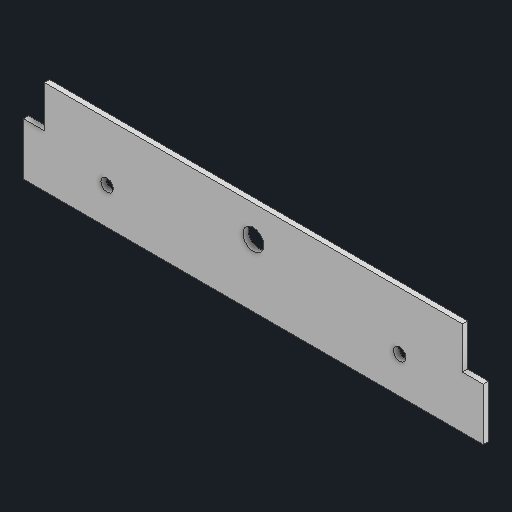
# Autodesk Inventor part: sUPORTE1
Saved by Autodesk Inventor 2026.2 (Build 302298010, 298A)
## iProperties
Created: 2026-02-20
Part Number: sUPORTE1
Material: Generic
Document SubType Name: Modeling
Designer: 062210040
Density: 1 g/cm^3
Appearance: Default
Author: 062210040
Autodesk Inventor part; units mm, degrees
ref_plane "YZ Plane" through (0, 0, 0) normal (1, 0, 0) x (0, 1, 0)
ref_plane "XZ Plane" through (0, 0, 0) normal (0, 1, 0) x (-1, 0, 0)
ref_plane "XY Plane" through (0, 0, 0) normal (0, 0, 1) x (1, 0, 0)
sketch "Sketch1" plane through (0, 0, 0) normal (0, 0, 1) x (1, 0, 0)
  line L0 (0, 0) -> (0, 50)
  line L1 (0, 50) -> (20, 50)
  line L2 (20, 50) -> (20, 90)
  line L3 (20, 90) -> (420, 90)
  line L4 (420, 90) -> (420, 50)
  line L5 (420, 50) -> (440, 50)
  line L6 (440, 50) -> (440, 0)
  line L7 (440, 0) -> (0, 0)
  circle A0 centre (220, 60) radius 10
  circle A1 centre (80, 35) radius 6
  circle A2 centre (360, 35) radius 6
  circle A3 centre (80, 35) radius 50
  circle A4 centre (130, 35) radius 6
  circle A5 centre (310, 35) radius 6
  dimension "d1" = 50
  dimension "d2" = 20
  dimension "d3" = 40
  dimension "d4" = 400
  dimension "d5" = 40
  dimension "d6" = 20
  dimension "d7" = 20
  dimension "d8" = 12
  dimension "d9" = 12
  dimension "d10" = 80
  dimension "d11" = 80
  dimension "d12" = 35
  dimension "d13" = 35
  dimension "d14" = 30
  dimension "d17" = 100
  dimension "d18" = 12
  dimension "d19" = 12
  dimension "d20" = 130
  dimension "d21" = 130
  dimension "d22" = 35
  dimension "d23" = 35
  constraints: 16 end point, 6 centre point, 5 perpendicular, 2 horizontal, 1 coincident, 1 vertical
  measures "d1" distance of L0.start L0.end
  measures "d2" distance of L0.end L1.end
  measures "d3" distance of L1.end L2.end
  measures "d4" distance of L2.end L3.end
  measures "d5" distance of L3.end L4.end
  measures "d6" distance of L4.end L5.end
  measures "d7" diameter of A0
  measures "d8" diameter of A1
  measures "d9" diameter of A2
  measures "d10" distance from line of L6 A2.centre
  measures "d11" distance from line of L0 A1.centre
  measures "d12" distance from line of L7 A1.centre
  measures "d13" distance from line of A2.centre L7
  measures "d14" distance from line of L3 A0.centre
  measures "d17" diameter of A3
  measures "d18" diameter of A4
  measures "d19" diameter of A5
  measures "d20" distance from line of L6 A5.centre
  measures "d21" distance from line of L0 A4.centre
  measures "d22" distance from line of L7 A4.centre
  measures "d23" distance from line of L7 A5.centre
extrude "Extrusion1" add sketch "Sketch1" along normal blind 5 contours L0 L1 L2 L3 L4 L5 L6 L7 A3 A4 | A3 A4 L7 | A4 A3 | A3 A4 | A5
body "Solid1"
